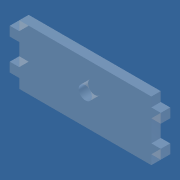
# Autodesk Inventor part: acrylic kinect plate
Saved by Autodesk Inventor 2012 (Build 160160000, 160)
## iProperties
Created: 2012-10-30
Part Number: acrylic kinect plate
Material: Default
Document SubType Name: Modeling
Designer: Ed
Density: 1 g/cm^3
Author: Ed
Autodesk Inventor part; units mm, degrees
ref_plane "YZ Plane" through (0, 0, 0) normal (1, 0, 0) x (0, 1, 0)
ref_plane "XZ Plane" through (0, 0, 0) normal (0, 1, 0) x (-1, 0, 0)
ref_plane "XY Plane" through (0, 0, 0) normal (0, 0, 1) x (1, 0, 0)
sketch "Sketch1" plane through (0, 0, 0) normal (0, 0, 1) x (1, 0, 0)
  line L0 (-44.45, 0) -> (44.45, 0)
  line L1 (44.45, 0) -> (44.45, 40)
  line L2 (44.45, 40) -> (-44.45, 40)
  line L3 (-44.45, 40) -> (-44.45, 0)
  line L4 (-50.8, 33.6525) -> (-44.45, 33.6525)
  line L5 (-44.45, 33.6525) -> (-44.45, 27.3025)
  line L6 (-44.45, 27.3025) -> (-50.8, 27.3025)
  line L7 (-50.8, 27.3025) -> (-50.8, 33.6525)
  line L8 (-50.8, 12.6975) -> (-44.45, 12.6975)
  line L9 (-44.45, 12.6975) -> (-44.45, 6.3475)
  line L10 (-44.45, 6.3475) -> (-50.8, 6.3475)
  line L11 (-50.8, 6.3475) -> (-50.8, 12.6975)
  line L12 (0, 40) -> (0, 32.8851)
  line L13 (-44.45, 12.6975) -> (-44.45, 27.3025)
  line L14 (50.8, 33.6525) -> (44.45, 33.6525)
  line L15 (44.45, 33.6525) -> (44.45, 27.3025)
  line L16 (44.45, 27.3025) -> (50.8, 27.3025)
  line L17 (50.8, 27.3025) -> (50.8, 33.6525)
  line L18 (50.8, 12.6975) -> (44.45, 12.6975)
  line L19 (44.45, 12.6975) -> (44.45, 6.3475)
  line L20 (44.45, 6.3475) -> (50.8, 6.3475)
  line L21 (50.8, 6.3475) -> (50.8, 12.6975)
  line L22 (44.45, 12.6975) -> (44.45, 27.3025)
  point P0 (0, 0)
  point P1 (-44.45, 20)
  point P2 (0, 0)
  point P3 (44.45, 20)
  dimension "d0" = 40
  dimension "d1" = 88.9
  dimension "d2" = 6.35
  dimension "d3" = 6.35
  dimension "d4" = 14.605
  constraints: 46 end point, 9 symmetric about line, 8 parallel, 4 midpoint, 3 horizontal, 3 perpendicular, 2 equal length, 2 point on line, 1 coincident
  measures "d0" distance of L2.end L0.start
  measures "d1" distance of L0.start L0.end
  measures "d2" distance of L6.end L4.start
  measures "d3" distance of L4.start L4.end
  measures "d4" distance between parallel lines of L6 L8
extrude "Extrusion1" add sketch "Sketch1" along normal blind 6.35
hole "Hole1" at (0, 20.0102, 6.35) direction (0, 0, -1) diameter 8.9916 end through all clearance for "Flat Head Machine Screw" size "M8" standard "Ansi Metric M Profile"
body "Solid1"
